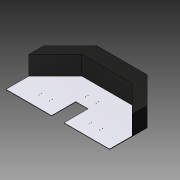
# Autodesk Inventor part: Charging Dock
Saved by Autodesk Inventor 2018 (Build 220112000, 112)
## iProperties
Created: 2017-03-09
Part Number: Charging Dock
Material: ABS Plastic
Document SubType Name: Modeling
Designer: Eightfold_Infotech
Density: 1.06 g/cm^3
Appearance: Smooth - White
Author: Eightfold_Infotech
Autodesk Inventor part; units mm, degrees
ref_plane "YZ Plane" through (0, 0, 0) normal (1, 0, 0) x (0, 1, 0)
ref_plane "XZ Plane" through (0, 0, 0) normal (0, 1, 0) x (-1, 0, 0)
ref_plane "XY Plane" through (0, 0, 0) normal (0, 0, 1) x (1, 0, 0)
sketch "Sketch2" plane through (0, 0, 0) normal (0, 1, 0) x (-1, 0, 0)
  line L0 (-200, -150) -> (200, -150)
  line L1 (200, -150) -> (200, -200)
  line L2 (-200, -200) -> (-200, -150)
  line L3 (0, -269.3547) -> (0, -73.2831)
  line L4 (200, -200) -> (200, -270)
  line L5 (200, -270) -> (-200, -270)
  line L6 (-200, -270) -> (-200, -200)
  line L7 (200, -150) -> (412.132, 62.132)
  line L8 (200, -150) -> (500, -150) construction
  line L9 (412.132, 62.132) -> (412.132, -57.868)
  line L10 (412.132, -57.868) -> (200, -270)
  line L11 (-200, -150) -> (-412.132, 62.132)
  line L12 (-412.132, 62.132) -> (-412.132, -57.868)
  line L13 (-412.132, -57.868) -> (-200, -270)
  point P0 (0, 0)
  point P1 (0, -175)
  point P2 (412.5, 61.0149)
  dimension "d9" = 400
  dimension "d10" = 50
  dimension "d39" = 70
  dimension "d40" = 200
  dimension "d41" = 45
  dimension "d42" = 120
  dimension "d43" = 150
  dimension "d51" = 300
  constraints: 28 end point, 3 perpendicular, 3 vertical, 2 horizontal, 2 symmetric about line, 1 equal length, 1 parallel
  measures "d9" distance of L1.end L2.start
  measures "d10" distance of L0.end L1.end
  measures "d39" distance of L1.end L4.end
  measures "d40" distance from line of L1 point (0, 0)
  measures "d41" angle of L8 L7
  measures "d42" distance of L7.end L9.end
  measures "d43" distance from line of point (0, 0) L0
  measures "d51" distance of L9.end L4.end
extrude "Extrusion2" add sketch "Sketch2" along normal blind 150
sketch "Sketch8" plane through (0, 0, 0) normal (0, -1, 0) x (1, 0, 0)
  line L0 (412.132, -57.868) -> (200, -270) projected
  line L1 (200, -270) -> (-200, -270) projected
  line L2 (-200, -270) -> (-412.132, -57.868) projected
  line L3 (-412.132, -57.868) -> (-412.132, 62.132) projected
  line L4 (-412.132, 62.132) -> (-200, -150) projected
  line L5 (-200, -150) -> (200, -150) projected
  line L6 (200, -150) -> (412.132, 62.132) projected
  line L7 (412.132, 62.132) -> (412.132, -57.868) projected
  line L8 (-412.132, 62.132) -> (-412.132, 242.132)
  line L9 (412.132, 62.132) -> (412.132, 242.132)
  line L10 (-412.132, 62.132) -> (-412.132, -57.868)
  line L11 (-412.132, -57.868) -> (-200, -270)
  line L12 (-200, -270) -> (200, -270)
  line L13 (200, -270) -> (412.132, -57.868)
  line L14 (412.132, -57.868) -> (412.132, 62.132)
  line L15 (50, 242.132) -> (50, 49.557)
  line L16 (50, 49.557) -> (-50, 49.557)
  line L17 (-50, 49.557) -> (-50, 242.132)
  line L18 (412.132, 242.132) -> (50, 242.132)
  line L19 (-50, 242.132) -> (-412.132, 242.132)
  dimension "d45" = 180
  dimension "d46" = 180
  dimension "d47" = 100
  constraints: 24 end point, 5 equal length, 1 point on line, 1 vertical
  measures "d45" distance of L3.end L8.end
  measures "d46" distance of L6.end L9.end
  measures "d47" distance of L15.end L16.end
extrude "Extrusion9" add sketch "Sketch8" along normal blind 4
sketch "Sketch9" plane through (0, -4, 0) normal (0, -1, 0) x (1, 0, 0)
  line L0 (200, -270) -> (-200, -270) projected
  line L1 (-200, -270) -> (-412.132, -57.868) projected
  line L2 (-412.132, -57.868) -> (-412.132, 242.132) projected
  line L3 (-412.132, 242.132) -> (-50, 242.132) projected
  line L4 (-50, 242.132) -> (-50, 49.557) projected
  line L5 (-50, 49.557) -> (50, 49.557) projected
  line L6 (50, 49.557) -> (50, 242.132) projected
  line L7 (50, 242.132) -> (412.132, 242.132) projected
  line L8 (412.132, 242.132) -> (412.132, -57.868) projected
  line L9 (412.132, -57.868) -> (200, -270) projected
  line L10 (200, -270) -> (-200, -270) projected
  line L11 (-200, -270) -> (-412.132, -57.868) projected
  line L12 (-412.132, -57.868) -> (-412.132, 242.132) projected
  line L13 (-412.132, 242.132) -> (-50, 242.132) projected
  line L14 (-50, 242.132) -> (-50, 49.557) projected
  line L15 (-50, 49.557) -> (50, 49.557) projected
  line L16 (50, 49.557) -> (50, 242.132) projected
  line L17 (50, 242.132) -> (412.132, 242.132) projected
  line L18 (412.132, 242.132) -> (412.132, -57.868) projected
  line L19 (412.132, -57.868) -> (200, -270) projected
  line L20 (200, -270) -> (-200, -270) projected
  line L21 (-200, -270) -> (-412.132, -57.868) projected
  line L22 (-412.132, -57.868) -> (-412.132, 242.132) projected
  line L23 (-412.132, 242.132) -> (-50, 242.132) projected
  line L24 (-50, 242.132) -> (-50, 49.557) projected
  line L25 (-50, 49.557) -> (50, 49.557) projected
  line L26 (50, 49.557) -> (50, 242.132) projected
  line L27 (50, 242.132) -> (412.132, 242.132) projected
  line L28 (412.132, 242.132) -> (412.132, -57.868) projected
  line L29 (412.132, -57.868) -> (200, -270) projected
  line L30 (250, 110) -> (250, 190) projected
  line L31 (200, -150) -> (412.132, 62.132) projected
  line L32 (-200, -150) -> (200, -150) projected
  line L33 (-412.132, 62.132) -> (-200, -150) projected
  line L34 (-412.132, 242.132) -> (-412.132, 62.132) projected
  line L35 (-50, 242.132) -> (-412.132, 242.132) projected
  line L36 (-50, 49.557) -> (-50, 242.132) projected
  line L37 (50, 49.557) -> (-50, 49.557) projected
  line L38 (50, 242.132) -> (50, 49.557) projected
  line L39 (412.132, 242.132) -> (50, 242.132) projected
  line L40 (412.132, 62.132) -> (412.132, 242.132) projected
  line L41 (200, -150) -> (412.132, 62.132) projected
  line L42 (-200, -150) -> (200, -150) projected
  line L43 (-412.132, 62.132) -> (-200, -150) projected
  line L44 (-412.132, 242.132) -> (-412.132, 62.132) projected
  line L45 (-50, 242.132) -> (-412.132, 242.132) projected
  line L46 (-50, 49.557) -> (-50, 242.132) projected
  line L47 (50, 49.557) -> (-50, 49.557) projected
  line L48 (50, 242.132) -> (50, 49.557) projected
  line L49 (412.132, 242.132) -> (50, 242.132) projected
  line L50 (412.132, 62.132) -> (412.132, 242.132) projected
  circle A0 centre (242.5, 150) radius 2
  circle A1 centre (242.5, 130) radius 2
  line L51 (200, 190) -> (200, 110) construction
  circle A2 centre (157.5, 150) radius 2
  circle A3 centre (157.5, 130) radius 2
  circle A4 centre (42.5, -20.443) radius 2
  circle A5 centre (42.5, -40.443) radius 2
  circle A6 centre (-42.5, -20.443) radius 2
  circle A7 centre (-42.5, -40.443) radius 2
  circle A8 centre (-157.5, 150) radius 2
  circle A9 centre (-157.5, 130) radius 2
  circle A10 centre (-242.5, 150) radius 2
  circle A11 centre (-242.5, 130) radius 2
  point P0 (0, 0)
  point P1 (0, 19.557)
  point P2 (-200, 190)
  dimension "d52" = 4
  dimension "d54" = 7.5
  dimension "d55" = 4
  dimension "d56" = 0
  dimension "d57" = 20
  dimension "d58" = 4
  dimension "d59" = 4
  dimension "d60" = 0
  dimension "d61" = 20
  dimension "d62" = 4
  dimension "d63" = 4
  dimension "d64" = 0
  dimension "d65" = 20
  constraints: 12 centre point, 2 end point, 2 symmetric about line, 2 other
  measures "d52" diameter of A0
  measures "d54" distance from line of L30 A0.centre
  measures "d55" diameter of A1
  measures "d56" horizontal distance of A0.centre A1.centre
  measures "d57" distance of A1.centre A0.centre
  measures "d58" diameter of A4
  measures "d59" diameter of A5
  measures "d60" horizontal distance of A4.centre A5.centre
  measures "d61" distance of A5.centre A4.centre
  measures "d62" diameter of A8
  measures "d63" diameter of A9
  measures "d64" horizontal distance of A8.centre A9.centre
  measures "d65" distance of A9.centre A8.centre
extrude "Extrusion10" cut sketch "Sketch9" against normal up to surface (4 mm away) contours A0 | A1 | A2 | A3 | A4 | A5 | A6 | A7 | A8 | A9 | A10 | A11
equation "\"d40\" = 0.5 * d9"
body "Solid1"
